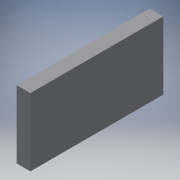
# Autodesk Inventor part: suporte
Saved by Autodesk Inventor 2016 (Build 200138000, 138)
## iProperties
Created: 2017-06-28
Part Number: suporte
Material: Genérico
Document SubType Name: Modeling
Designer: Fabio
Density: 1 g/cm^3
Appearance: Padrão
Author: Fabio
Autodesk Inventor part; units mm, degrees
ref_plane "YZ Plane" through (0, 0, 0) normal (1, 0, 0) x (0, 1, 0)
ref_plane "XZ Plane" through (0, 0, 0) normal (0, 1, 0) x (-1, 0, 0)
ref_plane "XY Plane" through (0, 0, 0) normal (0, 0, 1) x (1, 0, 0)
sketch "Esboço1" plane through (0, 0, 0) normal (1, 0, 0) x (0, 1, 0)
  line L0 (0.3875, 55) -> (-38.7875, 55)
  line L1 (-38.7875, 55) -> (-38.7875, -55)
  line L2 (-38.7875, -55) -> (38.7875, -55)
  line L3 (38.7875, -55) -> (0.3875, 55)
  point P0 (0, 0)
  point P1 (19.5875, 0)
  point P2 (0, -55)
  dimension "d4" = 77.575
  dimension "d5" = 110
  dimension "d6" = 39.175
  constraints: 8 end point, 2 midpoint, 1 horizontal, 1 horizontal alignment, 1 parallel, 1 perpendicular, 1 vertical alignment
  measures "d4" distance of L1.end L2.end
  measures "d5" distance of L0.end L1.end
  measures "d6" distance of L0.end L0.start
extrude "Extrusão1" add sketch "Esboço1" along normal blind 4
sketch "Esboço2" plane through (0, -38.7875, -55) normal (0, 0, -1) x (-1, 0, 0)
  line L0 (0, 0) -> (-4, 0) projected
  line L1 (0, 77.575) -> (-4, 77.575) projected
  line L2 (-4, 0) -> (-4, 77.575) projected
  line L3 (0, 39.175) -> (0, 0) projected
  line L4 (-4, 51.2875) -> (0, 51.2875)
  line L5 (0, 51.2875) -> (0, 26.2875)
  line L6 (0, 26.2875) -> (-4, 26.2875)
  line L7 (-4, 26.2875) -> (-4, 51.2875)
  point P0 (0, 38.7875)
  dimension "d7" = 77.575
  dimension "d8" = 25
  dimension "d9" = 26.2875
  constraints: 8 end point, 2 parallel, 2 point on line, 1 horizontal, 1 perpendicular
  measures "d7" distance between parallel lines of L0 L1
  measures "d8" distance of L4.end L5.end
  measures "d9" distance between parallel lines of L1 L4
extrude "Extrusão2" add sketch "Esboço2" along normal blind 4 contours L6 L2 L4 L5 L3
